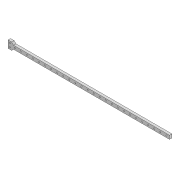
# Autodesk Inventor part: Test_feather
Saved by Autodesk Inventor 2022 (Build 260153000, 153)
## iProperties
Created: 2022-09-01
Part Number: Test_feather
Material: Generic
Document SubType Name: Modeling
Designer: dell
Density: 1 g/cm^3
Appearance: Default
Author: dell
Autodesk Inventor part; units mm, degrees
ref_plane "YZ Plane" through (0, 0, 0) normal (1, 0, 0) x (0, 1, 0)
ref_plane "XZ Plane" through (0, 0, 0) normal (0, 1, 0) x (-1, 0, 0)
ref_plane "XY Plane" through (0, 0, 0) normal (0, 0, 1) x (1, 0, 0)
sketch "Sketch1" plane through (0, 0, 0) normal (0, 0, 1) x (1, 0, 0)
  circle A0 centre (0, 0) radius 1.05
  circle A1 centre (0, 5.9) radius 1.05
  line L0 (-3, 8.95) -> (3, 8.95)
  line L1 (3, 8.95) -> (3, -3.05)
  line L2 (3, -3.05) -> (-3, -3.05)
  line L3 (-3, -3.05) -> (-3, 8.95)
  line L4 (3, 5.9) -> (263, 5.9)
  line L5 (263, 5.9) -> (263, 0)
  line L6 (263, 0) -> (3, 0)
  line L7 (3, 0) -> (3, 5.9)
  point P0 (3, 0)
  dimension "d0" = 2.1
  dimension "d1" = 2.1
  dimension "d2" = 5.9
  dimension "d3" = 3
  dimension "d4" = 3
  dimension "d5" = 12
  dimension "d6" = 3.05
  dimension "d7" = 260
  constraints: 16 end point, 4 parallel, 3 point on line, 2 centre point, 2 horizontal, 2 perpendicular, 1 coincident
  measures "d0" diameter of A0
  measures "d1" diameter of A1
  measures "d2" distance of point (0, 0) A1.centre
  measures "d3" distance from line of point (0, 0) L3
  measures "d4" distance from line of point (0, 0) L1
  measures "d5" distance between parallel lines of L0 L2
  measures "d6" distance from line of point (0, 0) L2
  measures "d7" distance between parallel lines of L1 L5
extrude "Extrusion1" add sketch "Sketch1" along normal blind 4
sketch "Sketch2" plane through (0, 0, 4) normal (0, 0, 1) x (1, 0, 0)
  circle A0 centre (8, 2.95) radius 1
  line L0 (-3, 8.95) -> (-3, -3.05) projected
  line L1 (3, 5.9) -> (3, 8.95) projected
  point P0 (0, 0)
  point P1 (-3, 2.95)
  dimension "d10" = 2
  dimension "d11" = 5
  constraints: 1 centre point, 1 horizontal alignment, 1 midpoint
  measures "d10" diameter of A0
  measures "d11" distance from line of L1 A0.centre
extrude "Extrusion2" cut sketch "Sketch2" against normal blind 10
pattern_linear "Rectangular Pattern1" count 26 spacing 10 along (1, 0, 0) of "Extrusion2"
chamfer "Chamfer1" distance 3 angle 45 2 edges at (3, 5.9, 2) (3, 0, 2)
body "Solid1"
